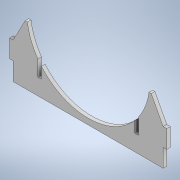
# Autodesk Inventor part: myDno
Saved by Autodesk Inventor 2022 (Build 260153000, 153)
## iProperties
Created: 2022-10-22
Part Number: myDno
Material: Типовые
Document SubType Name: Modeling
Designer: КозьминАндрей
Density: 1 g/cm^3
Appearance: По умолчанию
Author: КозьминАндрей
Autodesk Inventor part; units mm, degrees
ref_plane "YZ Plane" through (0, 0, 0) normal (1, 0, 0) x (0, 1, 0)
ref_plane "XZ Plane" through (0, 0, 0) normal (0, 1, 0) x (-1, 0, 0)
ref_plane "XY Plane" through (0, 0, 0) normal (0, 0, 1) x (1, 0, 0)
sketch "Эскиз1" plane through (0, 0, 0) normal (0, 0, 1) x (1, 0, 0)
  line L0 (-166, 74.5) -> (166, 74.5)
  line L1 (166, 74.5) -> (166, -74.5)
  line L2 (166, -74.5) -> (-166, -74.5)
  line L3 (-166, -74.5) -> (-166, 74.5)
  point P0 (0, 0)
  dimension "d0" = 332
  dimension "d1" = 149
  dimension "d3" = 166
  dimension "d4" = 74.5
  constraints: 8 end point, 2 parallel, 1 horizontal, 1 perpendicular
  measures "d0" distance of L1.end L2.end
  measures "d1" distance of L0.end L1.end
  measures "d3" distance from line of point (0, 0) L1
  measures "d4" distance from line of L0 point (0, 0)
extrude "Выдавливание1" add sketch "Эскиз1" along normal blind 8
sketch "Эскиз2" plane through (0, 0, 8) normal (0, 0, 1) x (1, 0, 0)
  line L0 (166, 74.5) -> (-166, 74.5) projected
  line L1 (-166, -74.5) -> (166, -74.5) projected
  circle A0 centre (0, 74.5) radius 136
  point P0 (0, 0)
  point P1 (-136, 74.5)
  point P2 (136, 74.5)
  dimension "d8" = 272
  constraints: 1 centre point, 1 midpoint
  measures "d8" diameter of A0
extrude "Выдавливание2" cut sketch "Эскиз2" against normal through all contours A0 L0 picked at (19.0214, 16.0372)
sketch "Эскиз3" plane through (0, 0, 8) normal (0, 0, 1) x (1, 0, 0)
  line L0 (103.5, -3.3701) -> (111.5, -3.3701)
  line L1 (111.5, -3.3701) -> (111.5, -38)
  line L2 (111.5, -38) -> (103.5, -38)
  line L3 (103.5, -38) -> (103.5, -3.3701)
  line L4 (-111.5, -3.3701) -> (-103.5, -3.3701)
  line L5 (-103.5, -3.3701) -> (-103.5, -38)
  line L6 (-103.5, -38) -> (-111.5, -38)
  line L7 (-111.5, -38) -> (-111.5, -3.3701)
  line L8 (166, -74.5) -> (166, 74.5) projected
  line L9 (-166, -74.5) -> (166, -74.5) projected
  line L10 (-166, 74.5) -> (-166, -74.5) projected
  arc A0 (-136, 74.5) -> (136, 74.5) centre (0, 74.5) ccw projected
  point P0 (0, 0)
  dimension "d11" = 54.5
  dimension "d12" = 36.5
  dimension "d13" = 54.5
  dimension "d14" = 36.5
  dimension "d15" = 8
  dimension "d16" = 8
  constraints: 16 end point, 4 parallel, 2 horizontal, 2 perpendicular, 1 point on circle, 1 point on line
  measures "d11" distance between parallel lines of L8 L1
  measures "d12" distance between parallel lines of L9 L2
  measures "d13" distance between parallel lines of L10 L7
  measures "d14" distance between parallel lines of L9 L6
  measures "d15" distance of L4.start L4.end
  measures "d16" distance of L0.start L0.end
extrude "Выдавливание3" cut sketch "Эскиз3" against normal through all
sketch "Эскиз4" plane through (-166, -74.5, 0) normal (-1, 0, 0) x (0, 0, 1)
  line L0 (0, 80) -> (8, 80)
  line L1 (8, 80) -> (8, 40)
  line L2 (8, 40) -> (0, 40)
  line L3 (0, 40) -> (0, 80)
  line L4 (0, 0) -> (8, 0) projected
  line L5 (0, 149) -> (0, 0) projected
  point P0 (0, 74.5)
  dimension "d19" = 40
  dimension "d20" = 40
  dimension "d21" = 8
  dimension "d22" = 0
  constraints: 8 end point, 2 parallel, 1 horizontal, 1 perpendicular
  measures "d19" distance between parallel lines of L2 L4
  measures "d20" distance of L0.end L1.end
  measures "d21" distance of L0.start L0.end
  measures "d22" distance between parallel lines of L5 L3
extrude "Выдавливание4" add sketch "Эскиз4" along normal blind 8
sketch "Эскиз5" plane through (166, -74.5, 0) normal (1, 0, 0) x (0, 0, -1)
  line L0 (-8, 80) -> (0, 80)
  line L1 (0, 80) -> (0, 40)
  line L2 (0, 40) -> (-8, 40)
  line L3 (-8, 40) -> (-8, 80)
  line L4 (0, 0) -> (-8, 0) projected
  line L5 (-8, 0) -> (-8, 149) projected
  point P0 (0, 74.5)
  dimension "d25" = 40
  dimension "d26" = 40
  dimension "d27" = 0
  dimension "d28" = 8
  constraints: 8 end point, 2 parallel, 1 horizontal, 1 perpendicular
  measures "d25" distance between parallel lines of L4 L2
  measures "d26" distance of L0.end L1.end
  measures "d27" distance between parallel lines of L5 L3
  measures "d28" distance of L1.end L2.end
extrude "Выдавливание5" add sketch "Эскиз5" along normal blind 8
sketch "Эскиз6" plane through (0, 0, 8) normal (0, 0, 1) x (1, 0, 0)
  line L0 (-136, 74.5) -> (-166, 74.5) projected
  line L1 (-166, 74.5) -> (-134.6663, 74.5)
  line L2 (-134.6663, 74.5) -> (-134.6663, 55.5)
  line L3 (-134.6663, 55.5) -> (-166, 55.5)
  line L4 (-166, 55.5) -> (-166, 74.5)
  line L5 (-166, 5.5) -> (-174, 5.5) projected
  arc A0 (-136, 74.5) -> (-111.5, -3.3701) centre (0, 74.5) ccw projected
  line L6 (166, 74.5) -> (136, 74.5) projected
  arc A1 (111.5, -3.3701) -> (136, 74.5) centre (0, 74.5) ccw projected
  line L7 (166, 74.5) -> (134.6663, 74.5)
  line L8 (134.6663, 74.5) -> (134.6663, 55.5)
  line L9 (134.6663, 55.5) -> (166, 55.5)
  line L10 (166, 55.5) -> (166, 74.5)
  line L11 (166, 5.5) -> (174, 5.5) projected
  point P0 (0, 0)
  dimension "d31" = 50
  dimension "d34" = 50
  constraints: 16 end point, 4 parallel, 2 horizontal, 2 perpendicular, 2 point on circle
  measures "d31" distance between parallel lines of L3 L5
  measures "d34" distance between parallel lines of L11 L9
extrude "Выдавливание6" cut sketch "Эскиз6" against normal through all contours A0 L3 L4 L0 | L10 L9 A1 L6
sketch "Эскиз7" plane through (0, 0, 8) normal (0, 0, 1) x (1, 0, 0)
  line L0 (-166, 55.5) -> (-166, 5.5) projected
  line L1 (-166, 55.5) -> (-134.6663, 55.5) projected
  line L2 (-166, 5.5) -> (-139.6663, 55.5)
  line L3 (-139.6663, 55.5) -> (-160.2816, 66.3576)
  line L4 (-160.2816, 66.3576) -> (-186.6153, 16.3576)
  line L5 (-186.6153, 16.3576) -> (-166, 5.5)
  line L6 (166, 5.5) -> (166, 55.5) projected
  line L7 (166, 5.5) -> (139.6663, 55.5)
  line L8 (139.6663, 55.5) -> (160.2816, 66.3576)
  line L9 (160.2816, 66.3576) -> (186.6153, 16.3576)
  line L10 (186.6153, 16.3576) -> (166, 5.5)
  line L11 (166, 55.5) -> (134.6663, 55.5) projected
  line L12 (139.6663, 55.5) -> (134.6663, 55.5)
  arc A0 (-134.6663, 55.5) -> (-111.5, -3.3701) centre (0, 74.5) ccw projected
  line L13 (-139.6663, 55.5) -> (-134.6663, 55.5)
  point P0 (0, 0)
  dimension "d35" = 5
  dimension "d36" = 5
  constraints: 20 end point, 4 parallel, 3 point on line, 2 perpendicular, 1 collinear, 1 horizontal
  measures "d35" distance of L1.end L2.end
  measures "d36" distance of L11.end L7.end
extrude "Выдавливание7" cut sketch "Эскиз7" against normal through all contours L1 L2 L0 | L7 L11 L6
